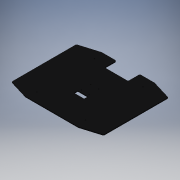
# Autodesk Inventor part: CoverPlate_CamMount
Saved by Autodesk Inventor 2016 (Build 200138000, 138)
## iProperties
Created: 2015-05-25
Part Number: CoverPlate_CamMount
Material: Generic
Document SubType Name: Modeling
Designer: Karl
Density: 1 g/cm^3
Appearance: Glossy - Black
Author: Karl
Autodesk Inventor part; units mm, degrees
ref_plane "YZ Plane" through (0, 0, 0) normal (1, 0, 0) x (0, 1, 0)
ref_plane "XZ Plane" through (0, 0, 0) normal (0, 1, 0) x (-1, 0, 0)
ref_plane "XY Plane" through (0, 0, 0) normal (0, 0, 1) x (1, 0, 0)
sketch "Sketch1" plane through (0, 0, 0) normal (0, 1, 0) x (-1, 0, 0)
  line L0 (149.225, -123.825) -> (-149.225, -123.825)
  line L1 (-149.225, -123.825) -> (-149.225, 123.825)
  line L2 (-149.225, 123.825) -> (149.225, 123.825)
  line L3 (149.225, 123.825) -> (149.225, -123.825)
  line L4 (149.225, -123.825) -> (-149.225, 123.825) construction
  line L5 (-149.225, -123.825) -> (149.225, 123.825) construction
  point P0 (0, 0)
  dimension "d0" = 298.45
  dimension "d1" = 247.65
  constraints: 12 end point, 2 midpoint, 2 parallel, 1 horizontal, 1 perpendicular
  measures "d0" distance of L1.end L2.end
  measures "d1" distance of L0.end L1.end
extrude "Extrusion1" add sketch "Sketch1" along normal blind 3.175
sketch "Sketch2" plane through (0, 3.175, 0) normal (0, 1, 0) x (1, 0, 0)
  line L0 (149.225, 123.825) -> (-149.225, 123.825) projected
  line L1 (-149.225, 123.825) -> (-149.225, -123.825) projected
  line L2 (-149.225, -123.825) -> (149.225, -123.825) projected
  line L3 (149.225, -123.825) -> (149.225, 123.825) projected
  line L4 (-149.225, 104.775) -> (-85.725, 123.825)
  line L5 (85.725, 123.825) -> (149.225, 104.775)
  line L6 (149.225, -104.775) -> (85.725, -123.825)
  line L7 (-85.725, -123.825) -> (-149.225, -104.775)
  point P0 (0, 0)
  dimension "d4" = 19.05
  dimension "d5" = 19.05
  dimension "d6" = 19.05
  dimension "d7" = 19.05
  dimension "d8" = 63.5
  dimension "d9" = 63.5
  dimension "d10" = 63.5
  constraints: 8 end point, 8 point on line, 1 parallel
  measures "d4" distance from line of L0 L4.start
  measures "d5" distance from line of L2 L7.end
  measures "d6" distance from line of L5.end L0
  measures "d7" distance from line of L2 L6.start
  measures "d8" distance from line of L1 L4.end
  measures "d9" distance from line of L3 L5.start
  measures "d10" distance from line of L1 L7.start
extrude "Extrusion2" cut sketch "Sketch2" against normal blind 3.175 contours L3 L5 L0 | L4 L1 L0 | L3 L2 L6 | L7 L2 L1
sketch "Sketch3" plane through (0, 3.175, 0) normal (0, 1, 0) x (1, 0, 0)
  line L0 (85.725, 123.825) -> (-85.725, 123.825) projected
  line L1 (-38.1, 123.825) -> (38.1, 123.825)
  line L2 (38.1, 123.825) -> (38.1, 85.725)
  line L3 (38.1, 85.725) -> (-38.1, 85.725)
  line L4 (-38.1, 85.725) -> (-38.1, 123.825)
  point P0 (0, 0)
  point P1 (0, 85.725)
  dimension "d13" = 38.1
  dimension "d14" = 76.2
  constraints: 8 end point, 2 parallel, 1 horizontal, 1 midpoint, 1 perpendicular, 1 point on line, 1 vertical alignment
  measures "d13" distance of L3.end L1.start
  measures "d14" distance of L2.end L3.end
extrude "Extrusion3" cut sketch "Sketch3" against normal blind 3.175
fillet "Fillet1" radius 3.175 12 edges at (38.1, 1.5875, -85.725) (-38.1, 1.5875, -85.725) (38.1, 1.5875, -123.825) (-38.1, 1.5875, -123.825) (85.725, 1.5875, -123.825) (-85.725, 1.5875, -123.825) (-149.225, 1.5875, -104.775) (149.225, 1.5875, -104.775) (-149.225, 1.5875, 104.775) (-85.725, 1.5875, 123.825) (85.725, 1.5875, 123.825) (149.225, 1.5875, 104.775)
sketch "Sketch4" plane through (0, 3.175, 0) normal (0, 1, 0) x (1, 0, 0)
  point P0 (0, 0)
  point P1 (-78.9686, 93.5863)
  point P2 (-78.9686, -93.5863)
  point P3 (78.9686, -93.5863)
  point P4 (78.9686, 93.5863)
  dimension "d18" = 93.5863
  dimension "d19" = 93.5863
  dimension "d20" = 78.9686
  dimension "d21" = 78.9686
  constraints: 2 horizontal alignment, 2 vertical alignment
  measures "d18" vertical distance of point (-78.969, -93.586) point (0, 0)
  measures "d19" vertical distance of point (-78.969, 93.586) point (0, 0)
  measures "d20" horizontal distance of point (-78.969, 93.586) point (0, 0)
  measures "d21" horizontal distance of point (78.969, 93.586) point (0, 0)
hole "Hole1" at (-78.9686, 3.175, -93.5863) at (-78.9686, 3.175, 93.5863) at (78.9686, 3.175, 93.5863) at (78.9686, 3.175, -93.5863) direction (0, -1, 0) diameter 3.302 end through all
sketch "Sketch5" plane through (0, 3.175, 0) normal (0, 1, 0) x (1, 0, 0)
  line L0 (-149.225, 102.4127) -> (-149.225, -102.4127) projected
  line L1 (149.225, -102.4127) -> (149.225, 102.4127) projected
  point P0 (0, 0)
  point P1 (-12.7, 15.24)
  point P2 (12.7, 15.24)
  point P3 (-12.7, -15.24)
  point P4 (12.7, -15.24)
  dimension "d38" = 25.4
  dimension "d39" = 25.4
  dimension "d40" = 30.48
  dimension "d44" = 15.24
  dimension "d45" = 15.24
  dimension "d46" = 12.7
  dimension "d47" = 12.7
  dimension "d48" = 12.7
  measures "d38" distance of point (12.7, 15.24) point (-12.7, 15.24)
  measures "d39" distance of point (-12.7, -15.24) point (12.7, -15.24)
  measures "d40" distance of point (12.7, -15.24) point (12.7, 15.24)
  measures "d44" vertical distance of point (0, 0) point (-12.7, 15.24)
  measures "d45" vertical distance of point (0, 0) point (12.7, 15.24)
  measures "d46" horizontal distance of point (0, 0) point (12.7, 15.24)
  measures "d47" horizontal distance of point (12.7, -15.24) point (0, 0)
  measures "d48" horizontal distance of point (-12.7, -15.24) point (0, 0)
hole "Hole3" at (-12.7, 3.175, -15.24) at (12.7, 3.175, -15.24) at (-12.7, 3.175, 15.24) at (12.7, 3.175, 15.24) direction (0, -1, 0) diameter 3.302 end through all
sketch "Sketch6" plane through (0, 3.175, 0) normal (0, 1, 0) x (1, 0, 0)
  line L0 (-16.51, -22.86) -> (16.51, -22.86)
  line L1 (16.51, -22.86) -> (16.51, -35.56)
  line L2 (16.51, -35.56) -> (-16.51, -35.56)
  line L3 (-16.51, -35.56) -> (-16.51, -22.86)
  point P0 (0, 0)
  dimension "d56" = 33.02
  dimension "d57" = 22.86
  dimension "d58" = 16.51
  dimension "d61" = 12.7
  constraints: 8 end point, 2 parallel, 1 horizontal, 1 perpendicular
  measures "d56" distance between parallel lines of L1 L3
  measures "d57" distance from line of point (0, 0) L0
  measures "d58" distance from line of L1 point (0, 0)
  measures "d61" distance of L0.end L1.end
extrude "Extrusion4" cut sketch "Sketch6" against normal blind 25.4
equation "\"d18\" = d19"
body "Solid1"
